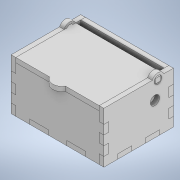
# Autodesk Inventor part: music box
Saved by Autodesk Inventor 2020 (Build 240168000, 168)
## iProperties
Created: 2021-11-21
Part Number: music box
Material: Generic
Document SubType Name: Modeling
Designer: rwte
Density: 1 g/cm^3
Appearance: Default
Author: rwte
Autodesk Inventor part; units mm, degrees
sketch "Sketch1" plane through (0, 0, 0) normal (0, 1, 0) x (-1, 0, 0)
  line L0 (30, -22.5) -> (-30, -22.5)
  line L1 (-30, -22.5) -> (-30, 22.5)
  line L2 (-30, 22.5) -> (30, 22.5)
  line L3 (30, 22.5) -> (30, -22.5)
  line L4 (30, -22.5) -> (-30, 22.5) construction
  line L5 (-30, -22.5) -> (30, 22.5) construction
  line L6 (-30, -22.5) -> (-27, -22.5)
  line L7 (-27, -22.5) -> (-27, -13.5)
  line L8 (-27, -13.5) -> (-30, -13.5)
  line L9 (-30, -13.5) -> (-30, -22.5)
  line L10 (42, 0) -> (-42, 0) projected
  line L11 (0, -31.5) -> (0, 31.5) projected
  line L12 (-30, -4.5) -> (-27, -4.5)
  line L13 (-27, -4.5) -> (-27, 4.5)
  line L14 (-27, 4.5) -> (-30, 4.5)
  line L15 (-30, 4.5) -> (-30, -4.5)
  line L16 (-30, 13.5) -> (-27, 13.5)
  line L17 (-27, 13.5) -> (-27, 22.5)
  line L18 (-27, 22.5) -> (-30, 22.5)
  line L19 (-30, 22.5) -> (-30, 13.5)
  line L20 (30, -22.5) -> (27, -22.5)
  line L21 (27, -22.5) -> (27, -13.5)
  line L22 (27, -13.5) -> (30, -13.5)
  line L23 (30, -13.5) -> (30, -22.5)
  line L24 (30, -4.5) -> (27, -4.5)
  line L25 (27, -4.5) -> (27, 4.5)
  line L26 (27, 4.5) -> (30, 4.5)
  line L27 (30, 4.5) -> (30, -4.5)
  line L28 (30, 13.5) -> (27, 13.5)
  line L29 (27, 13.5) -> (27, 22.5)
  line L30 (27, 22.5) -> (30, 22.5)
  line L31 (30, 22.5) -> (30, 13.5)
  line L32 (-6, 22.5) -> (6, 22.5)
  line L33 (6, 22.5) -> (6, 19.5)
  line L34 (6, 19.5) -> (-6, 19.5)
  line L35 (-6, 19.5) -> (-6, 22.5)
  line L36 (18, 22.5) -> (30, 22.5)
  line L37 (30, 22.5) -> (30, 19.5)
  line L38 (30, 19.5) -> (18, 19.5)
  line L39 (18, 19.5) -> (18, 22.5)
  line L40 (-18, 22.5) -> (-30, 22.5)
  line L41 (-30, 22.5) -> (-30, 19.5)
  line L42 (-30, 19.5) -> (-18, 19.5)
  line L43 (-18, 19.5) -> (-18, 22.5)
  line L44 (-30, -22.5) -> (30, -22.5)
  line L45 (-27, -22.5) -> (-30, -22.5)
  line L46 (27, -22.5) -> (30, -22.5)
  line L47 (-6, -22.5) -> (6, -22.5)
  line L48 (6, -22.5) -> (6, -19.5)
  line L49 (6, -19.5) -> (-6, -19.5)
  line L50 (-6, -19.5) -> (-6, -22.5)
  line L51 (18, -22.5) -> (30, -22.5)
  line L52 (30, -22.5) -> (30, -19.5)
  line L53 (30, -19.5) -> (18, -19.5)
  line L54 (18, -19.5) -> (18, -22.5)
  line L55 (-18, -22.5) -> (-30, -22.5)
  line L56 (-30, -22.5) -> (-30, -19.5)
  line L57 (-30, -19.5) -> (-18, -19.5)
  line L58 (-18, -19.5) -> (-18, -22.5)
  point P0 (0, 0)
  point P1 (27, -19.5)
  point P2 (30, -4.5)
  point P3 (30, 4.5)
  point P4 (27, 19.5)
  point P5 (6, 22.5)
  point P6 (-27, 19.5)
  point P7 (-30, 4.5)
  point P8 (-27, -19.5)
  point P9 (-18, -22.5)
  point P10 (-6, -22.5)
  point P11 (6, -22.5)
  dimension "d0" = 45
  dimension "d1" = 60
  dimension "d2" = 3
  dimension "d3" = 9
  dimension "d4" = 9
  dimension "d5" = 9
  dimension "d6" = 3
  dimension "d7" = 12
  dimension "d8" = 12
  constraints: 114 end point, 29 symmetric about line, 15 point on line, 14 parallel, 9 perpendicular, 7 collinear, 4 horizontal, 1 midpoint
  measures "d0" distance of L0.end L1.end
  measures "d1" distance of L0.start L0.end
  measures "d2" distance of L7.end L8.end
  measures "d3" distance of L6.end L7.end
  measures "d4" distance between parallel lines of L12 L8
  measures "d5" distance of L14.end L16.start
  measures "d6" distance of L42.end L40.start
  measures "d7" distance from line of L1.end L43
  measures "d8" distance between parallel lines of L43 L35
extrude "Extrusion1" add sketch "Sketch1" along normal blind 3 contours L0 L48 L49 L11 L10 L25 L24 L3 L22 L21 L53 L54 | L0 L58 L57 L7 L8 L1 L12 L13 L10 L11 L49 L50 | L26 L25 L10 L11 L34 L33 L2 L39 L38 L29 L28 L3 | L10 L13 L14 L1 L16 L17 L42 L43 L2 L35 L34 L11
ref_plane "Work Plane1" through (0, 0, 22.5) normal (0, 0, 1) x (1, 0, 0)
sketch "Sketch2" plane through (0, 0, 22.5) normal (0, 0, 1) x (1, 0, 0)
  line L0 (-30, 0) -> (-30, 3)
  line L1 (30, 0) -> (30, 3)
  line L2 (-30, 0) -> (-27, 0)
  line L3 (-27, 0) -> (-18, 0)
  line L4 (-18, 0) -> (-6, 0)
  line L5 (-6, 0) -> (6, 0)
  line L6 (6, 0) -> (18, 0)
  line L7 (18, 0) -> (27, 0)
  line L8 (27, 0) -> (30, 0)
  line L9 (-30, 0) -> (-30, 3)
  line L10 (-30, 0) -> (30, 0)
  line L11 (30, 0) -> (30, 30)
  line L12 (30, 30) -> (-30, 30)
  line L13 (-30, 30) -> (-30, 0)
  line L14 (-27, 0) -> (-18, 0)
  line L15 (-18, 0) -> (-18, 3)
  line L16 (-27, 3) -> (-18, 3)
  line L17 (-27, 0) -> (-27, 3)
  line L18 (-30, 0) -> (-27, 0)
  line L19 (-27, 0) -> (-27, 3)
  line L20 (-30, 3) -> (-27, 3)
  line L21 (-30, 0) -> (-30, 3)
  line L22 (-18, 0) -> (-6, 0)
  line L23 (-6, 0) -> (-6, 3)
  line L24 (-18, 3) -> (-6, 3)
  line L25 (-18, 0) -> (-18, 3)
  line L26 (-6, 0) -> (6, 0)
  line L27 (6, 0) -> (6, 3)
  line L28 (-6, 3) -> (6, 3)
  line L29 (-6, 0) -> (-6, 3)
  line L30 (6, 0) -> (18, 0)
  line L31 (18, 0) -> (18, 3)
  line L32 (6, 3) -> (18, 3)
  line L33 (6, 0) -> (6, 3)
  line L34 (18, 0) -> (27, 0)
  line L35 (27, 0) -> (27, 3)
  line L36 (18, 3) -> (27, 3)
  line L37 (18, 0) -> (18, 3)
  line L38 (27, 0) -> (30, 0)
  line L39 (30, 0) -> (30, 3)
  line L40 (27, 3) -> (30, 3)
  line L41 (27, 0) -> (27, 3)
  line L42 (-27, 0) -> (-30, 0)
  line L43 (-30, 0) -> (-18, 0)
  line L44 (-18, 0) -> (-18, 3)
  line L45 (-18, 3) -> (-30, 3)
  line L46 (-30, 3) -> (-30, 0)
  line L47 (6, 0) -> (-6, 0)
  line L48 (-6, 0) -> (6, 0)
  line L49 (6, 0) -> (6, 3)
  line L50 (6, 3) -> (-6, 3)
  line L51 (-6, 3) -> (-6, 0)
  line L52 (27, 0) -> (18, 0)
  line L53 (27, 0) -> (30, 0)
  line L54 (18, 0) -> (30, 0)
  line L55 (30, 0) -> (30, 3)
  line L56 (30, 3) -> (18, 3)
  line L57 (18, 3) -> (18, 0)
  line L58 (27, 0) -> (30, 0)
  line L59 (30, 0) -> (30, 6)
  line L60 (30, 6) -> (27, 6)
  line L61 (27, 6) -> (27, 0)
  line L62 (30, 12) -> (30, 18)
  line L63 (30, 18) -> (27, 18)
  line L64 (27, 18) -> (27, 12)
  line L65 (27, 12) -> (30, 12)
  line L66 (30, 24) -> (30, 30)
  line L67 (30, 30) -> (27, 30)
  line L68 (27, 30) -> (27, 24)
  line L69 (27, 24) -> (30, 24)
  line L70 (0, -6) -> (0, 36)
  line L71 (-30, 0) -> (-30, 3)
  line L72 (-27, 0) -> (-30, 0)
  line L73 (-30, 0) -> (-30, 30)
  line L74 (-27, 0) -> (-27, 3)
  line L75 (-27, 0) -> (-30, 0)
  line L76 (-30, 0) -> (-30, 3)
  line L77 (-27, 3) -> (-30, 3)
  line L78 (-27, 0) -> (-27, 3)
  line L79 (-27, 0) -> (-30, 0)
  line L80 (-30, 0) -> (-30, 3)
  line L81 (-27, 0) -> (-30, 0)
  line L82 (-30, 0) -> (-30, 6)
  line L83 (-30, 6) -> (-27, 6)
  line L84 (-27, 6) -> (-27, 0)
  line L85 (-30, 12) -> (-30, 18)
  line L86 (-30, 18) -> (-27, 18)
  line L87 (-27, 18) -> (-27, 12)
  line L88 (-27, 12) -> (-30, 12)
  line L89 (-30, 24) -> (-30, 30)
  line L90 (-30, 30) -> (-27, 30)
  line L91 (-27, 30) -> (-27, 24)
  line L92 (-27, 24) -> (-30, 24)
  point P0 (0, 0)
  point P1 (18, 0)
  point P2 (-6, 0)
  point P3 (6, 0)
  point P4 (27, 0)
  point P5 (-27, 30)
  point P6 (-30, 24)
  point P7 (-30, 18)
  point P8 (-30, 12)
  point P9 (-27, 3)
extrude "Extrusion2" add sketch "Sketch2" against normal blind 3 separate body contours L17 L16 L15 L3 | L13 L88 L87 L86 L92 L91 L12 L70 L28 L24 L16 L84 L83 | L23 L28 L70 L5 | L70 L28 L27 L5 | L70 L12 L68 L69 L11 L63 L64 L65 L60 L61 L36 L32 L28 | L31 L36 L35 L7
ref_plane "Work Plane2" through (30, 0, 0) normal (1, 0, 0) x (0, 1, 0)
sketch "Sketch3" plane through (30, 0, 0) normal (1, 0, 0) x (0, 1, 0)
  line L0 (0, 19.5) -> (0, 13.5)
  line L1 (0, 13.5) -> (3, 13.5)
  line L2 (3, 19.5) -> (3, 13.5)
  line L3 (0, 19.5) -> (3, 19.5)
  line L4 (0, 22.5) -> (6, 22.5)
  line L5 (0, 22.5) -> (0, 19.5)
  line L6 (6, 19.5) -> (0, 19.5)
  line L7 (6, 22.5) -> (6, 19.5)
  line L8 (0, 4.5) -> (0, -4.5)
  line L9 (0, -4.5) -> (3, -4.5)
  line L10 (3, 4.5) -> (3, -4.5)
  line L11 (0, 4.5) -> (3, 4.5)
  line L12 (0, -13.5) -> (0, -19.5)
  line L13 (0, -19.5) -> (3, -19.5)
  line L14 (3, -13.5) -> (3, -19.5)
  line L15 (0, -13.5) -> (3, -13.5)
  line L16 (0, -19.5) -> (0, -22.5)
  line L17 (0, -22.5) -> (3, -22.5)
  line L18 (3, -19.5) -> (3, -22.5)
  line L19 (0, -19.5) -> (3, -19.5)
  line L20 (12, 22.5) -> (18, 22.5)
  line L21 (12, 22.5) -> (12, 19.5)
  line L22 (18, 19.5) -> (12, 19.5)
  line L23 (18, 22.5) -> (18, 19.5)
  line L24 (24, 22.5) -> (30, 22.5)
  line L25 (24, 22.5) -> (24, 19.5)
  line L26 (30, 19.5) -> (24, 19.5)
  line L27 (30, 22.5) -> (30, 19.5)
  line L28 (18, 22.5) -> (24, 22.5)
  line L29 (6, 22.5) -> (12, 22.5)
  line L30 (0, 13.5) -> (0, 4.5)
  line L31 (0, -4.5) -> (0, -13.5)
  line L32 (0, 19.5) -> (0, 22.5)
  line L33 (0, 22.5) -> (30, 22.5)
  line L34 (30, 22.5) -> (30, -22.5)
  line L35 (30, -22.5) -> (0, -22.5)
  line L36 (0, -22.5) -> (0, 22.5)
  line L37 (18, 19.5) -> (24, 19.5)
  line L38 (24, 19.5) -> (24, 22.5)
  line L39 (24, 22.5) -> (33, 22.5)
  line L40 (33, 22.5) -> (33, 19.5)
  line L41 (33, 19.5) -> (24, 19.5)
  line L42 (12, 19.5) -> (18, 19.5)
  line L43 (18, 22.5) -> (12, 22.5)
  line L44 (12, 19.5) -> (12, 22.5)
  line L45 (12, 22.5) -> (24, 22.5)
  line L46 (24, 22.5) -> (24, 19.5)
  line L47 (24, 19.5) -> (12, 19.5)
  line L48 (0, 19.5) -> (0, 22.5)
  line L49 (0, 22.5) -> (0, 22.5)
  line L50 (0, 22.5) -> (0, 19.5)
  line L51 (0, 19.5) -> (0, 19.5)
  line L52 (3, 13.5) -> (3, 19.5)
  line L53 (3, 19.5) -> (3, 13.5)
  line L54 (3, 13.5) -> (0, 13.5)
  line L55 (0, 13.5) -> (0, 19.5)
  line L56 (0, 19.5) -> (3, 19.5)
  line L57 (3, -4.5) -> (3, 4.5)
  line L58 (0, 4.5) -> (3, 4.5)
  line L59 (3, 4.5) -> (3, -4)
  line L60 (3, -4) -> (0, -4)
  line L61 (0, -4) -> (0, 4.5)
  line L62 (0, -13.5) -> (3, -13.5)
  line L63 (3, -13.5) -> (3, -19.5)
  line L64 (3, -19.5) -> (0, -19.5)
  line L65 (0, -19.5) -> (0, -13.5)
  line L66 (0, -19.5) -> (3, -19.5)
  line L67 (3, -19.5) -> (3, -22.5)
  line L68 (0, -19.5) -> (3, -19.5)
  line L69 (3, -19.5) -> (3, -22.5)
  line L70 (3, -22.5) -> (0, -22.5)
  line L71 (0, -22.5) -> (0, -19.5)
  line L72 (24, 22.5) -> (24, 19.5)
  line L73 (24, 19.5) -> (24, 19.5)
  line L74 (6, 19.5) -> (0, 19.5)
  line L75 (12, 19.5) -> (6, 19.5)
  line L76 (3, 4.5) -> (3, 13.5)
  line L77 (3, 4.5) -> (3, 13.5)
  line L78 (3, -4.5) -> (3, -13.5)
  line L79 (-7.1, 0) -> (42.6, 0)
  line L80 (0, -19.5) -> (3, -19.5)
  line L81 (0, -22.5) -> (6, -22.5)
  line L82 (0, -22.5) -> (0, -19.5)
  line L83 (6, -19.5) -> (0, -19.5)
  line L84 (6, -22.5) -> (6, -19.5)
  line L85 (12, -22.5) -> (18, -22.5)
  line L86 (12, -22.5) -> (12, -19.5)
  line L87 (18, -19.5) -> (12, -19.5)
  line L88 (18, -22.5) -> (18, -19.5)
  line L89 (24, -22.5) -> (30, -22.5)
  line L90 (24, -22.5) -> (24, -19.5)
  line L91 (30, -19.5) -> (24, -19.5)
  line L92 (30, -22.5) -> (30, -19.5)
  line L93 (18, -22.5) -> (24, -22.5)
  line L94 (6, -22.5) -> (12, -22.5)
  line L95 (0, -19.5) -> (0, -22.5)
  line L96 (0, -22.5) -> (30, -22.5)
  line L97 (18, -19.5) -> (24, -19.5)
  line L98 (24, -19.5) -> (24, -22.5)
  line L99 (24, -22.5) -> (33, -22.5)
  line L100 (33, -22.5) -> (33, -19.5)
  line L101 (33, -19.5) -> (24, -19.5)
  line L102 (12, -19.5) -> (18, -19.5)
  line L103 (18, -22.5) -> (12, -22.5)
  line L104 (12, -19.5) -> (12, -22.5)
  line L105 (12, -22.5) -> (24, -22.5)
  line L106 (24, -22.5) -> (24, -19.5)
  line L107 (24, -19.5) -> (12, -19.5)
  line L108 (0, -19.5) -> (0, -22.5)
  line L109 (0, -22.5) -> (0, -22.5)
  line L110 (0, -22.5) -> (0, -19.5)
  line L111 (0, -19.5) -> (0, -19.5)
  line L112 (0, -19.5) -> (3, -19.5)
  line L113 (24, -22.5) -> (24, -19.5)
  line L114 (24, -19.5) -> (24, -19.5)
  line L115 (6, -19.5) -> (0, -19.5)
  line L116 (12, -19.5) -> (6, -19.5)
  line L117 (30, 22.5) -> (33, 22.5)
  line L118 (33, 22.5) -> (33, -22.5)
  line L119 (33, -22.5) -> (30, -22.5)
  line L120 (30, -22.5) -> (30, 22.5)
  circle A0 centre (31.5, -12.5) radius 4
  circle A1 centre (31.5, -12.5) radius 2.5
  line L121 (31.5, -22.5) -> (31.5, -12.5) construction
  point P0 (0, 0)
  point P1 (12, -22.5)
  point P2 (18, -22.5)
  point P3 (33, -16.2081)
  point P4 (33, -8.7919)
extrude "Extrusion3" add sketch "Sketch3" against normal blind 3 separate body contours L3 L2 L1 L0 | L5 L4 L7 L6 L3 | L6 L75 L22 L37 L26 L34 L79 L10 L76 L2 | L11 L10 L79 L8 | L79 L10 L60 L8 | L21 L20 L23 L22 | L79 L34 A0 L91 L97 L87 L116 L83 L14 L78 L10 | L60 L10 L9 L8 | L79 L118 A0 L34 | L34 L41 L118 L79 | L25 L24 L27 L26 | L27 L39 L40 L41 | A0 L118 A1 L34 | L34 A1 A0 | L15 L14 L13 L12 | A0 L118 A1 | A0 L118 L101 L34 | L34 A1 L118 A0 | L13 L18 L17 L16 | L83 L84 L35 L18 | L101 L100 L99 L34 | L34 L35 L90 L91 | L87 L88 L35 L86
mirror "Mirror1" about plane through (0, 0, 0) normal (1, 0, 0) of "Extrusion3" bodies 3
ref_plane "Work Plane3" through (0, 0, -22.5) normal (0, 0, 1) x (1, 0, 0)
sketch "Sketch4" plane through (0, 0, -22.5) normal (0, 0, 1) x (1, 0, 0)
  line L0 (-27, 12) -> (-27, 18) projected
  line L1 (-27, 18) -> (-30, 18) projected
  line L2 (-30, 18) -> (-30, 24) projected
  line L3 (-30, 24) -> (-27, 24) projected
  line L4 (-27, 24) -> (-27, 30) projected
  line L5 (-27, 30) -> (27, 30) projected
  line L6 (27, 30) -> (27, 24) projected
  line L7 (27, 24) -> (30, 24) projected
  line L8 (30, 24) -> (30, 18) projected
  line L9 (30, 18) -> (27, 18) projected
  line L10 (27, 18) -> (27, 12) projected
  line L11 (27, 12) -> (30, 12) projected
  line L12 (30, 12) -> (30, 6) projected
  line L13 (30, 6) -> (27, 6) projected
  line L14 (27, 6) -> (27, 0) projected
  line L15 (27, 0) -> (18, 0) projected
  line L16 (18, 0) -> (18, 3) projected
  line L17 (18, 3) -> (6, 3) projected
  line L18 (6, 3) -> (6, 0) projected
  line L19 (6, 0) -> (-6, 0) projected
  line L20 (-6, 0) -> (-6, 3) projected
  line L21 (-6, 3) -> (-18, 3) projected
  line L22 (-18, 3) -> (-18, 0) projected
  line L23 (-18, 0) -> (-27, 0) projected
  line L24 (-27, 0) -> (-27, 6) projected
  line L25 (-27, 6) -> (-30, 6) projected
  line L26 (-30, 6) -> (-30, 12) projected
  line L27 (-30, 12) -> (-27, 12) projected
  line L28 (27, 3) -> (18, 3) projected
  line L29 (6, 3) -> (-6, 3) projected
  line L30 (-18, 3) -> (-27, 3) projected
  line L31 (-27, 12) -> (-27, 6) projected
  line L32 (-27, 24) -> (-27, 18) projected
  line L33 (27, 24) -> (27, 18) projected
  line L34 (27, 12) -> (27, 6) projected
  line L35 (-27, 0) -> (-27, 3) projected
  line L36 (27, 3) -> (-27, 3)
  line L37 (-27, 3) -> (-27, 48)
  line L38 (27, 30) -> (27, 3)
  line L39 (-27, 18) -> (-27, 24) projected
  line L40 (-27, 24) -> (-30, 24)
  line L41 (-30, 24) -> (-30, 18)
  line L42 (-30, 18) -> (-27, 18)
  line L43 (-27, 18) -> (-27, 24)
  line L44 (-27, 6) -> (-27, 12) projected
  line L45 (-27, 12) -> (-30, 12)
  line L46 (-30, 12) -> (-30, 6)
  line L47 (-30, 6) -> (-27, 6)
  line L48 (-27, 6) -> (-27, 12)
  line L49 (-27, 0) -> (-30, 0) projected
  line L50 (-18, 3) -> (-27, 3)
  line L51 (-27, 3) -> (-27, 0)
  line L52 (-27, 0) -> (-18, 0)
  line L53 (-18, 0) -> (-18, 3)
  line L54 (6, 3) -> (-6, 3)
  line L55 (-6, 3) -> (-6, 0)
  line L56 (-6, 0) -> (6, 0)
  line L57 (6, 0) -> (6, 3)
  line L58 (18, 0) -> (18, 3) projected
  line L59 (27, 3) -> (18, 3)
  line L60 (18, 3) -> (18, 0)
  line L61 (18, 0) -> (27, 0)
  line L62 (27, 0) -> (27, 3)
  line L63 (30, 6) -> (30, 12) projected
  line L64 (27, 6) -> (30, 6)
  line L65 (30, 6) -> (30, 12)
  line L66 (30, 12) -> (27, 12)
  line L67 (27, 12) -> (27, 6)
  line L68 (27, 18) -> (27, 24) projected
  line L69 (27, 18) -> (30, 18)
  line L70 (30, 18) -> (30, 24)
  line L71 (30, 24) -> (27, 24)
  line L72 (27, 24) -> (27, 18)
  line L73 (30, 33) -> (27, 33) projected
  line L74 (-30, 33) -> (-27, 33) projected
  line L75 (27, 33) -> (-27, 33)
  line L76 (27, 29) -> (27, 34) projected
  line L77 (27, 30) -> (27, 33)
  point P0 (0, 0)
  point P1 (-27, 30)
  dimension "d22" = 45
  constraints: 66 end point, 15 parallel, 11 perpendicular, 7 horizontal, 1 point on line
  measures "d22" distance of L30.end L37.end
extrude "Extrusion4" add sketch "Sketch4" along normal blind 3 separate body
ref_plane "Work Plane4" through (0, 31.5, 0) normal (0, 1, 0) x (-1, 0, 0)
sketch "Sketch7" plane through (0, 31.5, 0) normal (0, 1, 0) x (-1, 0, 0)
  line L0 (-27, -22.5) -> (-27, -19.5) projected
  line L1 (27, 19.5) -> (-27, 19.5)
  line L2 (-27, 19.5) -> (-27, -16.2081)
  line L3 (27, -16.2081) -> (27, 19.5)
  line L4 (27, 19.5) -> (-27, -19.5) construction
  line L5 (-27, 19.5) -> (18.0784, -13.0566) construction
  line L6 (27, 19.5) -> (18, 19.5) projected
  line L7 (27, 19.5) -> (-27, 19.5)
  line L8 (-27, 19.5) -> (-27, 22.5)
  line L9 (-27, 22.5) -> (27, 22.5)
  line L10 (27, 22.5) -> (27, 19.5)
  line L11 (-27, 13.5) -> (-27, 22.5) projected
  line L12 (27, -4.5) -> (27, 4.5) projected
  line L13 (27, -14.4) -> (27, -10.6)
  line L14 (27, -10.6) -> (30, -10.6)
  line L15 (30, -10.6) -> (30, -14.4)
  line L16 (30, -14.4) -> (27, -14.4)
  line L17 (-27, 4.5) -> (-27, -4.5) projected
  line L18 (-27, 4.9108) -> (-27, -1.8809)
  line L19 (-27, -1.8809) -> (-30, -1.8809)
  line L20 (-30, -1.8809) -> (-30, 4.9108)
  line L21 (-30, 4.9108) -> (-27, 4.9108)
  line L22 (30, -15) -> (27, -15) projected
  line L23 (27, -10) -> (27, -15) projected
  line L24 (30, -15) -> (30, -10) projected
  line L25 (-27, -10) -> (-27, -15) projected
  line L26 (-30, -15) -> (-30, -10) projected
  line L27 (-27, -15) -> (-30, -15) projected
  line L28 (-27, -10) -> (-30, -10) projected
  line L29 (-27, -10) -> (-27, -15) projected
  line L30 (27, -10) -> (27, -15) projected
  line L31 (30, -10) -> (27, -10) projected
  line L32 (0, -32.1) -> (0, 35.1) projected
  line L33 (-27, -14.4) -> (-27, -10.6)
  line L34 (-27, -10.6) -> (-30, -10.6)
  line L35 (-30, -10.6) -> (-30, -14.4)
  line L36 (-30, -14.4) -> (-27, -14.4)
  line L37 (-30, -15) -> (-27, -15)
  line L38 (-27, -10) -> (-27, -15)
  line L39 (-30, -15) -> (-30, -10)
  line L40 (-27, -10) -> (-27, -15)
  line L41 (-30, -10) -> (-27, -10)
  line L42 (6, 19.5) -> (-6, 19.5) projected
  arc A0 (6, 19.5) -> (-6, 19.5) centre (0, 19.5) ccw
  line L43 (30, -16.2081) -> (27, -16.2081) projected
  line L44 (-30, -16.2081) -> (-27, -16.2081) projected
  line L45 (27, -16.2081) -> (-27, -16.2081)
  point P0 (0, 0)
  point P1 (27, -12.5)
  point P2 (-27, -12.5)
  point P3 (-30, -10.6)
  point P4 (-30, -14.4)
  point P5 (-5.1962, 22.5)
  point P6 (5.1962, 22.5)
  dimension "d38" = 3
  dimension "d39" = 3
  dimension "d41" = 3.8
  dimension "d44" = 6
  constraints: 54 end point, 13 symmetric about line, 8 point on line, 7 parallel, 5 perpendicular, 4 midpoint, 2 point on circle, 1 centre point, 1 collinear, 1 horizontal
  measures "d38" distance of L13.end L14.end
  measures "d39" distance of L18.end L19.end
  measures "d41" distance of L14.end L15.end
  measures "d44" radius of A0
extrude "Extrusion7" add sketch "Sketch7" along normal mid plane 3 separate body contours L3 L45 L32 L1 | L1 A0 L9 L10 | L1 L32 L9 A0 | L9 L32 A0 | L32 L45 L2 L1 | L1 A0 L9 L32 | L9 A0 L32 | L1 L8 L9 A0 | L14 L15 L16 L3 | L36 L26 L34 L2
sketch "Sketch8" plane through (30, 0, 0) normal (1, 0, 0) x (0, 0, -1)
  line L0 (4.5, 3) -> (13.5, 3) projected
  line L1 (-13.5, 3) -> (-4.5, 3) projected
  line L2 (-19.5, 3) -> (-13.5, 3) projected
  line L3 (-19.5, 6) -> (-19.5, 0) projected
  line L4 (-19.5, 12) -> (-19.5, 6) projected
  line L5 (-19.5, 18) -> (-19.5, 12) projected
  line L6 (-19.5, 24) -> (-19.5, 18) projected
  line L7 (-19.5, 30) -> (-19.5, 24) projected
  line L8 (19.5, 24) -> (19.5, 33) projected
  line L9 (19.5, 18) -> (19.5, 24) projected
  line L10 (19.5, 12) -> (19.5, 18) projected
  line L11 (19.5, 6) -> (19.5, 12) projected
  line L12 (-19.5, 12) -> (-19.5, 6) projected
  line L13 (-19.5, 6) -> (-22.5, 6) projected
  line L14 (-22.5, 6) -> (-22.5, 0) projected
  line L15 (-22.5, 0) -> (-13.5, 0) projected
  line L16 (-13.5, 0) -> (-13.5, 3) projected
  line L17 (-13.5, 3) -> (-4.5, 3) projected
  line L18 (-4.5, 3) -> (-4.5, 0) projected
  line L19 (-4.5, 0) -> (4.5, 0) projected
  line L20 (4.5, 0) -> (4.5, 3) projected
  line L21 (4.5, 3) -> (13.5, 3) projected
  line L22 (13.5, 3) -> (13.5, 0) projected
  line L23 (13.5, 0) -> (22.5, 0) projected
  line L24 (22.5, 0) -> (22.5, 6) projected
  line L25 (22.5, 6) -> (19.5, 6) projected
  line L26 (19.5, 6) -> (19.5, 12) projected
  line L27 (19.5, 12) -> (22.5, 12) projected
  line L28 (22.5, 12) -> (22.5, 18) projected
  line L29 (22.5, 18) -> (19.5, 18) projected
  line L30 (19.5, 18) -> (19.5, 24) projected
  line L31 (19.5, 24) -> (22.5, 24) projected
  line L32 (22.5, 24) -> (22.5, 33) projected
  line L33 (22.5, 33) -> (16.2081, 33) projected
  arc A0 (16.2081, 33) -> (8.7919, 33) centre (12.5, 31.5) ccw projected
  line L34 (8.7919, 33) -> (-22.5, 33) projected
  line L35 (-22.5, 33) -> (-22.5, 24) projected
  line L36 (-22.5, 24) -> (-19.5, 24) projected
  line L37 (-19.5, 24) -> (-19.5, 18) projected
  line L38 (-19.5, 18) -> (-22.5, 18) projected
  line L39 (-22.5, 18) -> (-22.5, 12) projected
  line L40 (-22.5, 12) -> (-19.5, 12) projected
  circle A1 centre (12.5, 31.5) radius 2.5 projected
  line L41 (19.5, 0) -> (19.5, 6) projected
  line L42 (13.5, 3) -> (19.5, 3) projected
  point P0 (0, 0)
  point P1 (0, 3)
  point P2 (10.5, 21)
  dimension "d45" = 18
  dimension "d46" = 30
  measures "d45" vertical distance of L2.start point (10.5, 21)
  measures "d46" horizontal distance of point (10.5, 21) L2.start
hole "Hole1" at (30, 21, -10.5) direction (-1, 0, 0) diameter 6 depth 3 bodies 3
equation "\"d0\" = z"
equation "\"d1\" = x"
equation "\"d2\" = th"
equation "\"d4\" = d3"
equation "\"d5\" = d3"
equation "\"d6\" = th"
equation "\"d8\" = d7"
equation "\"d9\" = th"
equation "\"d13\" = th"
equation "\"d38\" = th"
equation "\"d39\" = th"
equation "\"x\" = 60"
equation "\"z\" = 45"
equation "\"th\" = 3"
equation "\"d11\" = 0.5 * z"
equation "\"d15\" = th"
equation "\"d17\" = d16"
equation "\"d21\" = -0.5 * z"
equation "\"d25\" = y + 0.5 * th"
equation "\"d33\" = th"
equation "\"d16\" = 6"
equation "\"y\" = 30"
body "Solid1"
body "Solid2"
body "Solid3"
body "Solid4"
body "Solid5"
